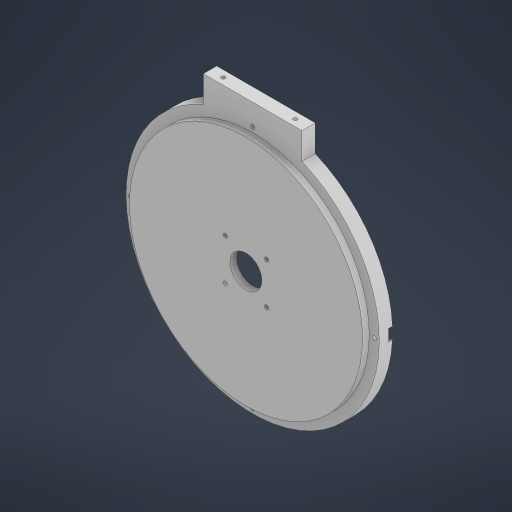
# Autodesk Inventor part: Motor Holder
Saved by Autodesk Inventor 2023 (Build 270158000, 158)
## iProperties
Created: 2023-04-06
Part Number: Motor Holder
Material: Generic
Document SubType Name: Modeling
Designer: vatdu
Density: 1 g/cm^3
Appearance: Default
Author: vatdu
Autodesk Inventor part; units mm, degrees
ref_plane "YZ Plane" through (0, 0, 0) normal (1, 0, 0) x (0, 1, 0)
ref_plane "XZ Plane" through (0, 0, 0) normal (0, 1, 0) x (-1, 0, 0)
ref_plane "XY Plane" through (0, 0, 0) normal (0, 0, 1) x (1, 0, 0)
sketch "Sketch1" plane through (0, 0, 0) normal (0, 0, 1) x (1, 0, 0)
  circle A0 centre (0, 0) radius 95
  dimension "d0" = 190
  constraints: 1 centre point, 1 coincident
  measures "d0" diameter of A0
extrude "Extrusion1" add sketch "Sketch1" along normal blind 10
sketch "Sketch2" plane through (0, 0, 10) normal (0, 0, 1) x (1, 0, 0)
  circle A0 centre (0, 0) radius 87.5
  dimension "d4" = 175
  constraints: 1 centre point, 1 coincident
  measures "d4" diameter of A0
extrude "Extrusion2" cut sketch "Sketch2" against normal blind 10
extrude "Extrusion3" add sketch "Sketch2" along normal blind 5
sketch "Sketch3" plane through (0, 0, 15) normal (0, 0, 1) x (1, 0, 0)
  line L0 (0, 0) -> (41, 0) construction
  line L1 (23.5, -23.5) -> (-23.5, -23.5)
  line L2 (-23.5, -23.5) -> (-23.5, 23.5)
  line L3 (-23.5, 23.5) -> (23.5, 23.5)
  line L4 (23.5, 23.5) -> (23.5, -23.5)
  line L5 (23.5, 0) -> (23.5, -23.5)
  circle A0 centre (15.5, -15.5) radius 1.5
  circle A1 centre (15.5, 15.5) radius 1.5
  circle A2 centre (-15.5, -15.5) radius 1.5
  circle A3 centre (-15.5, 15.5) radius 1.5
  circle A4 centre (0, 0) radius 12
  dimension "d13" = 47
  dimension "d14" = 47
  dimension "d15" = 23.5
  dimension "d16" = 23.5
  dimension "d34" = 3
  dimension "d35" = 24
  constraints: 12 end point, 5 centre point, 2 coincident, 2 horizontal, 2 parallel, 1 perpendicular, 1 point on line
  measures "d13" distance of L2.end L3.end
  measures "d14" distance of L1.end L2.end
  measures "d15" distance of L0.start L5.start
  measures "d16" distance of L5.start L5.end
  measures "d34" diameter of A0
  measures "d35" diameter of A4
extrude "Extrusion8" cut sketch "Sketch3" against normal blind 10 contours A0 | A1 | A2 | A3 | A4
sketch "Sketch8" plane through (0, 0, 10) normal (0, 0, 1) x (1, 0, 0)
  circle A0 centre (0, 0) radius 87.5 projected
  line L0 (0, 87.5) -> (-36.9939, 87.5)
  line L1 (0, 87.5) -> (36.9939, 87.5) construction
  line L2 (-36.9939, 87.5) -> (36.9939, 87.5)
  line L3 (36.9939, 87.5) -> (36.9939, 107.5)
  line L4 (36.9939, 107.5) -> (-36.9939, 107.5)
  line L5 (-36.9939, 107.5) -> (-36.9939, 87.5)
  dimension "d44" = 180
  dimension "d45" = 20
  constraints: 12 end point, 3 horizontal, 2 parallel, 1 collinear, 1 perpendicular, 1 vertical alignment, 1 other
  measures "d44" angle of L0 L1
  measures "d45" distance of L3.end L2.end
extrude "Extrusion10" cut sketch "Sketch8" against normal blind 10 contours L0 L5 L4 L3 L2
extrude "Extrusion11" add sketch "Sketch8" against normal blind 10 contours L0 L5 L4 L3 L2
sketch "Sketch6" plane through (0, 0, 0) normal (0, 0, -1) x (-1, 0, 0)
  circle A0 centre (0, -91.5) radius 1.5
  circle A1 centre (-91.5, 0) radius 1.5
  circle A2 centre (0, 91.5) radius 1.5
  circle A3 centre (91.5, 0) radius 1.5
  point P0 (0, 0)
  dimension "d26" = 3
  dimension "d27" = 3
  dimension "d28" = 3
  dimension "d29" = 3
  constraints: 4 centre point
  measures "d26" diameter of A0
  measures "d27" diameter of A1
  measures "d28" diameter of A2
  measures "d29" diameter of A3
extrude "Extrusion7" cut sketch "Sketch6" against normal blind 70
sketch "Sketch7" plane through (0, 0, 0) normal (0, 0, -1) x (-1, 0, 0)
  circle A0 centre (91.5, 0) radius 1.5 projected
  circle A1 centre (91.5, 0) radius 5.5
  circle A2 centre (0, -91.5) radius 1.5 projected
  circle A3 centre (0, -91.5) radius 5.5
  circle A4 centre (-91.5, 0) radius 1.5 projected
  circle A5 centre (-91.5, 0) radius 5.5
  circle A6 centre (0, 91.5) radius 1.5 projected
  circle A7 centre (0, 91.5) radius 5.5
  point P0 (0, 0)
  dimension "d38" = 11
  dimension "d39" = 11
  dimension "d40" = 11
  dimension "d41" = 11
  constraints: 4 centre point, 4 coincident
  measures "d38" diameter of A1
  measures "d39" diameter of A3
  measures "d40" diameter of A5
  measures "d41" diameter of A7
extrude "Extrusion9" cut sketch "Sketch7" against normal blind 3 contours A0 | A1 | A2 | A3 | A4 | A5 | A6 | A7
sketch "Sketch9" plane through (-36.9939, 107.5, 10) normal (0, 1, 0) x (1, 0, 0)
  line L0 (0, 0) -> (0, 10) projected
  line L1 (0, 5) -> (10, 5)
  line L2 (73.9879, 0) -> (73.9879, 10) projected
  line L3 (73.9879, 5) -> (63.9879, 5)
  circle A0 centre (10, 5) radius 1.5
  circle A1 centre (63.9879, 5) radius 1.5
  point P0 (36.9939, 10)
  dimension "d50" = 10
  dimension "d51" = 10
  dimension "d52" = 3
  dimension "d53" = 3
  constraints: 4 end point, 2 centre point, 2 coincident, 2 horizontal, 2 midpoint
  measures "d50" distance of L1.start L1.end
  measures "d51" distance of L3.start L3.end
  measures "d52" diameter of A0
  measures "d53" diameter of A1
extrude "Extrusion12" cut sketch "Sketch9" against normal blind 10
body "Solid1"
